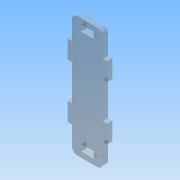
# Autodesk Inventor part: Back_Wall
Saved by Autodesk Inventor 2016 (Build 200138000, 138)
## iProperties
Created: 2015-06-25
Part Number: Back_Wall
Material: Generic
Document SubType Name: Modeling
Designer: Openlab
Density: 1 g/cm^3
Appearance: Polycarbonate - Clear
Author: Openlab
Autodesk Inventor part; units mm, degrees
ref_plane "YZ Plane" through (0, 0, 0) normal (1, 0, 0) x (0, 1, 0)
ref_plane "XZ Plane" through (0, 0, 0) normal (0, 1, 0) x (-1, 0, 0)
ref_plane "XY Plane" through (0, 0, 0) normal (0, 0, 1) x (1, 0, 0)
sketch "Sketch1" plane through (0, 0, 0) normal (0, 1, 0) x (-1, 0, 0)
  line L0 (8.5, -19.9274) -> (8.5, -42.3236) construction
  line L1 (13.2323, -33.5) -> (6.4845, -33.5) construction
  line L2 (17, -13.5) -> (19.45, -13.5)
  line L3 (19.45, -13.5) -> (19.45, -23.5)
  line L4 (19.45, -23.5) -> (17, -23.5)
  line L5 (17, -43.5) -> (19.45, -43.5)
  line L6 (19.45, -43.5) -> (19.45, -53.5)
  line L7 (19.45, -53.5) -> (17, -53.5)
  line L8 (0, -13.5) -> (-2.45, -13.5)
  line L9 (-2.45, -13.5) -> (-2.45, -23.5)
  line L10 (-2.45, -23.5) -> (0, -23.5)
  line L11 (0, -43.5) -> (-2.45, -43.5)
  line L12 (-2.45, -53.5) -> (0, -53.5)
  line L13 (-2.45, -53.5) -> (-2.45, -43.5)
  line L14 (17, -13.5) -> (17, -3)
  line L15 (17, -64) -> (17, -53.5)
  line L16 (17, -43.5) -> (17, -23.5)
  line L17 (0, -3) -> (0, -13.5)
  line L18 (0, -23.5) -> (0, -43.5)
  line L19 (0, -53.5) -> (0, -64)
  line L20 (14, 0) -> (3, 0)
  line L21 (3, -67) -> (14, -67)
  line L22 (12, -3) -> (5, -3)
  line L23 (5, -3) -> (5, -6.5)
  line L24 (5, -6.5) -> (12, -6.5)
  line L25 (12, -6.5) -> (12, -3)
  line L26 (12, -60.5) -> (5, -60.5)
  line L27 (5, -60.5) -> (5, -64)
  line L28 (5, -64) -> (12, -64)
  line L29 (12, -64) -> (12, -60.5)
  arc A0 (17, -3) -> (14, 0) centre (14, -3) ccw
  arc A1 (3, 0) -> (0, -3) centre (3, -3) ccw
  arc A2 (14, -67) -> (17, -64) centre (14, -64) ccw
  arc A3 (0, -64) -> (3, -67) centre (3, -64) ccw
  point P0 (0, 0)
  dimension "d8" = 10
  dimension "d9" = 20
  dimension "d17" = 2.45
  dimension "d21" = 67
  dimension "d22" = 17
  dimension "d23" = 7
  dimension "d24" = 3.5
  dimension "d25" = 3
  dimension "d27" = 6
  constraints: 60 end point, 15 parallel, 14 perpendicular, 12 point on line, 8 point on circle, 8 tangent, 6 horizontal, 5 collinear, 4 centre point, 3 equal length, 3 equal radius, 1 vertical, 6 other
  measures "d8" distance of L2.end L3.end
  measures "d9" distance between parallel lines of L5 L4
  measures "d17" distance of L8.start L8.end
  measures "d21" distance between parallel lines of L21 L20
  measures "d22" distance between parallel lines of L18 L16
  measures "d23" distance of L23.end L24.end
  measures "d24" distance of L24.end L22.start
  measures "d25" distance between parallel lines of L21 L28
  measures "d27" diameter of A1
extrude "Extrusion1" add sketch "Sketch1" along normal blind 3
body "Solid1"
